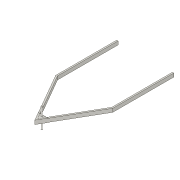
# Autodesk Inventor part: Hauling_Wishbone
Saved by Autodesk Inventor 2018 (Build 220112000, 112)
## iProperties
Created: 2017-08-21
Part Number: Hauling_Wishbone
Material: Generic
Document SubType Name: Modeling
Designer: thoma
Density: 1 g/cm^3
Appearance: Steel
Author: thoma
Autodesk Inventor part; units mm, degrees
ref_plane "YZ Plane" through (0, 0, 0) normal (1, 0, 0) x (0, 1, 0)
ref_plane "XZ Plane" through (0, 0, 0) normal (0, 1, 0) x (-1, 0, 0)
ref_plane "XY Plane" through (0, 0, 0) normal (0, 0, 1) x (1, 0, 0)
sketch "Sketch1" plane through (0, 0, 0) normal (0, 1, 0) x (-1, 0, 0)
  line L0 (0, 0) -> (0, 1079.8577)
  line L1 (0, 1079.8577) -> (990.6, -635.9118)
  line L2 (990.6, -635.9118) -> (990.6, -2844.8)
  line L3 (990.6, -2844.8) -> (1041.4, -2844.8)
  line L4 (1041.4, -2844.8) -> (1041.4, -622.3)
  line L5 (1041.4, -622.3) -> (0, 1181.4577)
  line L6 (0, 1181.4577) -> (-1041.4, -622.3)
  line L7 (-1041.4, -622.3) -> (-1041.4, -2844.8)
  line L8 (-1041.4, -2844.8) -> (-990.6, -2844.8)
  line L9 (-990.6, -2844.8) -> (-990.6, -635.9118)
  line L10 (-990.6, -635.9118) -> (0, 1079.8577)
  line L11 (0, 1079.8577) -> (0, 1181.4577)
  dimension "d0" = 2082.8
  dimension "d1" = 50.8
  dimension "d3" = 150
  dimension "d4" = 622.3
  dimension "d5" = 50.8
  dimension "d21" = 2222.5
  constraints: 24 end point, 3 equal length, 3 parallel, 3 perpendicular, 3 vertical, 2 point on line
  measures "d0" distance of L7.end L3.end
  measures "d1" distance between parallel lines of L4 L2
  measures "d3" angle of L1 L2
  measures "d4" vertical distance of L4.end L0.start
  measures "d5" distance between parallel lines of L5 L1
  measures "d21" distance of L3.end L4.end
extrude "Extrusion1" add sketch "Sketch1" against normal blind 127
sketch "Sketch2" plane through (0, 0, 0) normal (0, 1, 0) x (1, 0, 0)
  line L0 (-1041.4, 622.3) -> (0, -1181.4577) projected
  line L1 (-175.9764, -876.6577) -> (175.9764, -876.6577)
  line L2 (1041.4, 622.3) -> (0, -1181.4577) projected
  line L3 (175.9764, -876.6577) -> (0, -1181.4577)
  line L4 (0, -1181.4577) -> (-175.9764, -876.6577)
  line L5 (0, -1079.8577) -> (-990.6, 635.9118) projected
  point P0 (0, 0)
  dimension "d8" = 304.8
  constraints: 6 end point, 2 point on line, 1 collinear, 1 horizontal, 1 parallel
  measures "d8" distance from line of L0.end L1
extrude "Extrusion2" add sketch "Sketch2" along normal blind 6.35
sketch "Sketch3" plane through (0, -127, 0) normal (0, -1, 0) x (1, 0, 0)
  line L0 (-1041.4, -622.3) -> (-175.9764, 876.6577) projected
  line L1 (117.3176, 876.6577) -> (175.9764, 876.6577) projected
  line L2 (-175.9764, 876.6577) -> (175.9764, 876.6577)
  line L3 (1041.4, -622.3) -> (0, 1181.4577) projected
  line L4 (175.9764, 876.6577) -> (0, 1181.4577)
  line L5 (0, 1181.4577) -> (-175.9764, 876.6577)
  point P0 (0, 0)
  constraints: 6 end point, 1 collinear, 1 horizontal
extrude "Extrusion3" add sketch "Sketch3" along normal blind 6.35
sketch "Sketch4" plane through (0, 6.35, 0) normal (0, 1, 0) x (1, 0, 0)
  circle A0 centre (0, -927.4577) radius 25.4
  line L0 (0, -927.4577) -> (0, -876.6577)
  line L1 (117.3176, -876.6577) -> (-117.3176, -876.6577) projected
  point P0 (0, 0)
  dimension "d13" = 50.8
  dimension "d14" = 50.8
  constraints: 2 end point, 1 centre point, 1 midpoint, 1 vertical
  measures "d13" diameter of A0
  measures "d14" distance of L0.start L0.end
extrude "Extrusion4" add sketch "Sketch4" along normal blind 304.8
sketch "Sketch5" plane through (0, -133.35, 0) normal (0, -1, 0) x (1, 0, 0)
  line L0 (175.9764, 876.6577) -> (-175.9764, 876.6577) projected
  line L1 (0, 876.6577) -> (0, 927.4577)
  circle A0 centre (0, 927.4577) radius 25.4
  point P0 (0, 0)
  dimension "d17" = 50.8
  dimension "d18" = 50.8
  constraints: 2 end point, 1 centre point, 1 coincident, 1 midpoint, 1 vertical
  measures "d17" distance of L1.start L1.end
  measures "d18" diameter of A0
extrude "Extrusion5" add sketch "Sketch5" along normal blind 273.05
body "Solid1"
